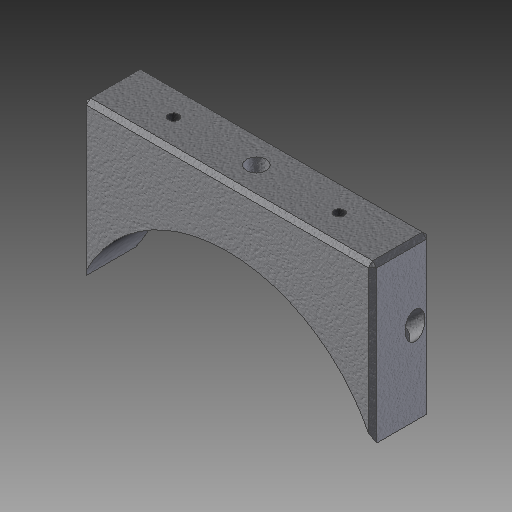
# Autodesk Inventor part: 1137_RU Mechanical Connector_V1
Saved by Autodesk Inventor 2020 (Build 240168000, 168)
## iProperties
Created: 2019-04-17
Part Number: 1137_RU Mechanical Connector_V1
Material: Generic
Document SubType Name: Modeling
Designer: e22ma
Density: 1 g/cm^3
Appearance: Coarse Textured - White
Mass: 158.049 g
Surface Area: 267.414 cm^2
Volume: 158.049 cm^3
Author: e22ma
Autodesk Inventor part; units mm, degrees
ref_plane "Work Plane1" through (0, 0, 0) normal (0, 0, 1) x (1, 0, 0)
sketch "Sketch1" plane through (0, 0, 0) normal (0, 0, 1) x (1, 0, 0)
  circle A0 centre (50.6671, 69.7373) radius 2.489 construction
  circle A1 centre (81.9811, 26.6373) radius 2.489 construction
  circle A2 centre (81.9811, -26.6373) radius 2.489 construction
  circle A3 centre (50.6671, -69.7373) radius 2.489 construction
  circle A4 centre (0, -86.2) radius 2.489 construction
  circle A5 centre (-50.6671, -69.7373) radius 2.489 construction
  circle A6 centre (-81.9811, -26.6373) radius 2.489 construction
  circle A7 centre (-81.9811, 26.6373) radius 2.489 construction
  circle A8 centre (-50.6671, 69.7373) radius 2.489 construction
  circle A9 centre (0, 86.2) radius 2.489 construction
  circle A10 centre (0, 0) radius 76.2 construction
  circle A11 centre (0, 0) radius 96.2 construction
  line L0 (129.3474, 57.0797) -> (-42.7255, 134.7715) construction
  line L1 (107.1095, 67.1202) -> (-20.4876, 124.731)
  line L2 (-20.4876, 124.731) -> (-51.4093, 56.2453)
  line L3 (-51.4093, 56.2453) -> (76.1878, -1.3655) construction
  line L4 (76.1878, -1.3655) -> (107.1095, 67.1202)
  arc A12 (76.1878, -1.3655) -> (-51.4093, 56.2453) centre (0, 0) ccw
  point P0 (0, 0)
  dimension "d0" = 140
  constraints: 8 end point, 4 point on circle, 2 parallel, 2 point on line, 1 centre point, 1 concentric, 1 perpendicular
  measures "d0" distance of L2.end L3.end
extrude "Extrusion1" add sketch "Sketch1" along normal blind 28
sketch "Sketch4" plane through (0, 0, 28) normal (0, 0, 1) x (1, 0, 0)
  line L0 (107.1095, 67.1202) -> (-20.4876, 124.731) projected
  line L1 (-20.4876, 124.731) -> (-51.4093, 56.2453) projected
  arc A0 (76.1878, -1.3655) -> (-51.4093, 56.2453) centre (0, 0) ccw projected
  line L2 (76.1878, -1.3655) -> (107.1095, 67.1202) projected
  line L3 (0, 0) -> (43.3109, 95.9256)
  line L4 (0, 0) -> (-26.9355, 71.2806)
  dimension "d5" = 45
  constraints: 4 end point, 1 coincident, 1 midpoint, 1 point on circle
  measures "d5" angle of L3 L4
ref_plane "Work Plane2" through (-26.9355, 71.2806, 28) normal (0.353484, -0.9354406, 0) x (0.9354406, 0.353484, 0)
sketch "Sketch6" plane through (-26.9355, 71.2806, 28) normal (0.353484, -0.9354406, 0) x (0.9354406, 0.353484, 0)
  line L0 (0, -13) -> (0, -28)
  point P0 (0, -20.5)
  dimension "d33" = 7.5
  constraints: 2 end point, 1 midpoint, 1 vertical
  measures "d33" distance of L0.end point (0, -20.5)
hole "Hole1" at (-26.9355, 71.2806, 7.5) direction (-0.353484, 0.9354406, 0) diameter 3.264 end through all clearance for "Flat Head Machine Screw (82)" size "#4" standard "Ansi Unified Screw Threads"
ref_plane "Work Plane3" through (-37.1865, 98.4083, 28) normal (0.353484, -0.9354406, 0) x (0.9354406, 0.353484, 0)
sketch "Sketch7" plane through (-37.1865, 98.4083, 28) normal (0.353484, -0.9354406, 0) x (0.9354406, 0.353484, 0)
  circle A0 centre (0, -20.5) radius 1.632 projected
  point P0 (0, -28)
  constraints: 1 coincident
hole "Hole2" at (-37.1865, 98.4083, 7.5) direction (0.353484, -0.9354406, 0) diameter 3.264 end through all counterbore diameter 9.525 counterbore depth 18 clearance for "Hex Machine Screw" size "#4" standard "Ansi Unified Screw Threads"
ref_plane "Work Plane4" through (12.3893, 27.4399, 0) normal (-0.9114073, 0.4115055, 0) x (0, 0, 1)
mirror "Mirror1" about plane through (12.3893, 27.4399, 0) normal (-0.9114073, 0.4115055, 0) of "Hole2", "Hole1"
sketch "Sketch8" plane through (-20.4876, 124.731, 28) normal (0.4115055, 0.9114073, 0) x (0.9114073, -0.4115055, 0)
  line L0 (0, 28) -> (0, 0) projected
  line L1 (140, 28) -> (140, 0) projected
  line L2 (0, 28) -> (0, 0) projected
  line L3 (0, 14) -> (140, 14)
  point P0 (70, 28)
  point P1 (30, 14)
  point P2 (110, 14)
  dimension "d21" = 30
  dimension "d22" = 30
  constraints: 2 end point, 2 midpoint, 2 point on line
  measures "d21" distance from line of L0 point (30, 14)
  measures "d22" distance from line of L1 point (110, 14)
hole "Hole3" at (6.8547, 112.3858, 14) at (79.7672, 79.4654, 14) direction (-0.4115055, -0.9114073, 0) diameter 4.978 end through all thread size "1/4-20 UNC" class "2B" standard "ANSI Unified Screw Threads"
chamfer "Chamfer1" distance 2 angle 45 8 edges at (-35.9484, 90.4881, 28) (43.3109, 95.9256, 28) (-20.4876, 124.731, 14) (-35.9484, 90.4881, 0) (43.3109, 95.9256, 0) (107.1095, 67.1202, 14) (91.6486, 32.8774, 28) (91.6486, 32.8774, 0)
sketch "Sketch9" plane through (-18.6647, 123.908, 26) normal (0.4115055, 0.9114073, 0) x (0.9114073, -0.4115055, 0)
  line L0 (0, 0) -> (0, 24) projected
  line L1 (136, 24) -> (136, 0) projected
  line L2 (0, 12) -> (136, 12)
  point P0 (68, 26)
  point P1 (68, 12)
  constraints: 3 midpoint, 2 end point
hole "Hole4" at (43.3109, 95.9256, 14) direction (-0.4115055, -0.9114073, 0) diameter 3.264 end through all counterbore diameter 9.525 counterbore depth 20 clearance for "Hex Machine Screw" size "#4" standard "Ansi Unified Screw Threads"
body "Solid1"
